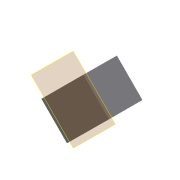
# Autodesk Inventor part: ServoHolder
Saved by Autodesk Inventor 2018 (Build 220112000, 112)
## iProperties
Created: 2018-10-26
Part Number: ServoHolder
Material: Generic
Document SubType Name: Modeling
Designer: Vulnic
Density: 1 g/cm^3
Appearance: Default
Author: Vulnic
Autodesk Inventor part; units mm, degrees
ref_plane "YZ Plane" through (0, 0, 0) normal (1, 0, 0) x (0, 1, 0)
ref_plane "XZ Plane" through (0, 0, 0) normal (0, 1, 0) x (-1, 0, 0)
ref_plane "XY Plane" through (0, 0, 0) normal (0, 0, 1) x (1, 0, 0)
ref_plane "Work Plane1" through (-120.5056, -67.4861, 19.6827) normal (0, -1, 0) x (-0.7095338, 0, -0.7046714)
sketch "Sketch1" plane through (-120.5056, -67.4861, 19.6827) normal (0, -1, 0) x (-0.7095338, 0, -0.7046714)
  line L0 (-3.5869, -1.5817) -> (38.9131, -1.5817)
  line L1 (38.9131, -1.5817) -> (38.9131, 24.4183)
  line L2 (38.9131, 24.4183) -> (-3.5869, 24.4183)
  line L3 (-3.5869, 24.4183) -> (-3.5869, -1.5817)
  point P0 (-71.6329, 98.8824)
  dimension "d0" = 42.5
  dimension "d1" = 26
  constraints: 8 end point, 2 parallel, 1 horizontal, 1 perpendicular
  measures "d0" distance of L1.end L2.end
  measures "d1" distance of L0.end L1.end
extrude "Extrusion1" add sketch "Sketch1" against normal blind 24
shell "Shell1" thickness 6 removed faces 1 at (-129.1269, -59.4861, 13.3497)
sketch "Sketch2" plane through (-119.0751, -67.4861, 23.3326) normal (-0.7046714, 0, 0.7095338) x (0.7095338, 0, 0.7046714)
  line L0 (0, 0) -> (-42.5, 0) projected
  line L1 (-42.5, 0) -> (-42.5, 24) projected
  line L2 (0, 0) -> (-42.5, 0)
  line L3 (-42.5, 0) -> (-42.5, 5)
  line L4 (-42.5, 5) -> (0, 5)
  line L5 (0, 5) -> (0, 0)
  line L6 (0, 24) -> (-42.5, 24)
  line L7 (-42.5, 24) -> (-42.5, 19)
  line L8 (-42.5, 19) -> (0, 19)
  line L9 (0, 19) -> (0, 24)
  point P0 (68.046, 67.4861)
  dimension "d5" = 5
  dimension "d7" = 5
  constraints: 16 end point, 4 parallel, 2 horizontal, 2 perpendicular, 2 point on line
  measures "d5" distance of L4.end L0.start
  measures "d7" distance of L8.end L6.start
extrude "Extrusion2" cut sketch "Sketch2" against normal through all
sketch "Sketch3" plane through (-119.0751, -62.4861, 23.3326) normal (0, -1, 0) x (-0.7095338, 0, -0.7046714)
  line L0 (42.5, 26) -> (42.5, 0) projected
  line L1 (0, 26) -> (42.5, 26)
  line L2 (42.5, 26) -> (42.5, 21)
  line L3 (42.5, 21) -> (0, 21)
  line L4 (0, 21) -> (0, 26)
  point P0 (-68.046, 100.4641)
  dimension "d10" = 5
  constraints: 8 end point, 2 parallel, 1 horizontal, 1 perpendicular, 1 point on line
  measures "d10" distance of L3.end L1.start
extrude "Extrusion3" cut sketch "Sketch3" against normal through all
body "Solid1"
